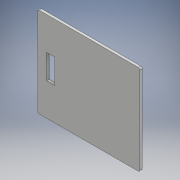
# Autodesk Inventor part: PalingAtasFix
Saved by Autodesk Inventor 2017 (Build 210142000, 142)
## iProperties
Created: 2019-05-10
Part Number: PalingAtasFix
Material: Generic
Document SubType Name: Modeling
Designer: Faiz
Density: 1 g/cm^3
Appearance: Default
Author: Faiz
Autodesk Inventor part; units mm, degrees
ref_plane "YZ Plane" through (0, 0, 0) normal (1, 0, 0) x (0, 1, 0)
ref_plane "XZ Plane" through (0, 0, 0) normal (0, 1, 0) x (-1, 0, 0)
ref_plane "XY Plane" through (0, 0, 0) normal (0, 0, 1) x (1, 0, 0)
sketch "Sketch1" plane through (0, 0, 0) normal (0, 1, 0) x (-1, 0, 0)
  line L0 (60.5, 55) -> (-60.5, 55)
  line L1 (-62.5, 53) -> (-62.5, -53)
  line L2 (-60.5, -55) -> (60.5, -55)
  line L3 (62.5, -53) -> (62.5, 53)
  arc A0 (62.5, 53) -> (60.5, 55) centre (60.5, 53) ccw
  arc A1 (60.5, -55) -> (62.5, -53) centre (60.5, -53) ccw
  arc A2 (-62.5, -53) -> (-60.5, -55) centre (-60.5, -53) ccw
  arc A3 (-60.5, 55) -> (-62.5, 53) centre (-60.5, 53) ccw
  point P0 (0, 0)
  constraints: 8 end point, 8 point on circle, 8 tangent, 4 centre point, 3 equal radius, 2 parallel, 1 horizontal, 1 perpendicular
extrude "Extrusion1" add sketch "Sketch1" along normal mid plane 3
sketch "Sketch2" plane through (0, 1.5, 0) normal (0, 1, 0) x (1, 0, 0)
  line L0 (8.4973, 37.5) -> (-31.5027, 37.5)
  line L1 (-31.5027, 37.5) -> (-31.5027, -37.5)
  line L2 (-31.5027, -37.5) -> (8.4973, -37.5)
  line L3 (8.4973, -37.5) -> (8.4973, 37.5)
  line L4 (8.4973, 37.5) -> (48.4973, 37.5)
  line L5 (48.4973, 37.5) -> (48.4973, -37.5)
  line L6 (48.4973, -37.5) -> (8.4973, -37.5)
  line L7 (-41.3593, 15) -> (-51.3593, 15)
  line L8 (-51.3593, 15) -> (-51.3593, -15)
  line L9 (-51.3593, -15) -> (-41.3593, -15)
  line L10 (-41.3593, -15) -> (-41.3593, 15)
  point P0 (0, 0)
  constraints: 22 end point, 4 parallel, 2 horizontal, 2 perpendicular, 2 symmetric about line
extrude "Extrusion2" cut sketch "Sketch2" against normal blind 3 contours L10 L9 L8 L7
body "Solid1"
